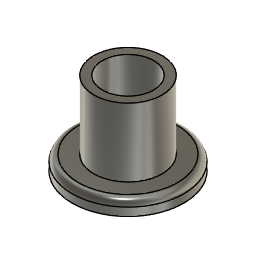
M6x8 socket head sleeve cap v3 (Autodesk Fusion 360 design; units mm, degrees)
Autodesk Fusion 360 part; units mm, degrees
sketch "Sketch1" plane through (0, 0, 0) normal (0, 0, 1) x (1, 0, 0)
  circle A0 centre (0, 0) radius 4
  circle A1 centre (0, 0) radius 3
  circle A2 centre (0, 0) radius 6.55
  dimension "d1" = 8
  dimension "d2" = 6
  dimension "d3" = 13.1
  constraint coincident A0.centre A1.centre
  constraint concentric A0 A2
  measures "d1" diameter of A0
  measures "d2" diameter of A1
  measures "d3" diameter of A2
extrude "Extrude1" add sketch "Sketch1" along normal blind 2.7 makes body 1 at (6.5419, -0.3265, 1.8) makes body 2 at (2.9963, -0.1495, 1.8)
extrude "Extrude2" add 1 faces at (-1.1591, 0.5829, 2.7) along direction (0, 0, 1) blind 1.3 on bodies 2 bodies 2
extrude "Extrude3" add sketch "Sketch1" along normal blind 10.7 contours A0 bodies 1 2
sketch "Sketch2" plane through (0, 0, 0) normal (0, 0, -1) x (1, 0, 0)
  circle A0 centre (0, 0) radius 6.55
  line L0 (-2, 0) -> (2, 0) construction
  line L1 (1, -1.7321) -> (-1, 1.7321) construction
  line L2 (1, 1.7321) -> (-1, -1.7321) construction
  line L3 (-2, -2.5) -> (-2, 2.5) construction
  line L4 (-2, 2.5) -> (2, 2.5) construction
  line L5 (2, 2.5) -> (2, -2.5) construction
  line L6 (2, -2.5) -> (-2, -2.5) construction
  line L7 (-1, -1.7321) -> (-2, -1.1547) construction
  line L8 (-1, 1.7321) -> (-2, 1.1547) construction
  line L9 (-2, -1.1547) -> (-2, 1.1547)
  line L10 (1, -1.7321) -> (2, -1.1547) construction
  line L11 (1, 1.7321) -> (2, 1.1547) construction
  line L12 (-2, -1.1547) -> (0, -2.3094)
  line L13 (0, -2.3094) -> (2, -1.1547)
  line L14 (2, 1.1547) -> (0, 2.3094)
  line L15 (0, 2.3094) -> (-2, 1.1547)
  line L16 (2, -1.1547) -> (2, 1.1547)
  dimension "d10" = 4
  dimension "d12" = 360
  constraint horizontal L0
  constraint midpoint A0.centre L0
  constraint vertical L3
  constraint perpendicular L3 L4
  constraint perpendicular L4 L5
  constraint perpendicular L5 L6
  constraint coincident L3 L7.end
  constraint perpendicular L2 L7
  constraint coincident L3 L8.end
  constraint perpendicular L1 L8
  constraint coincident L5 L10.end
  constraint perpendicular L1 L10
  constraint coincident L5 L11.end
  constraint perpendicular L2 L11
  constraint parallel L7 L12
  constraint perpendicular L1 L13
  constraint perpendicular L2 L14
  constraint parallel L8 L15
  measures "d10" distance of L0.start L0.end
extrude "Extrude4" cut sketch "Sketch2" against normal blind 2 contours L9 L12 L13 L14 L15 L16 bodies 1
chamfer "Chamfer1" distance 0.5 distance2 1.9 6 edges at (-1, 1.7321, 2) (1, 1.7321, 2) (2, 0, 2) (1, -1.7321, 2) (-2, 0, 2) (-1, -1.7321, 2) measured on face at (-1.3333, 1.5396, 0.6667) measured on face at (0.6667, 1.9245, 0.6667) measured on face at (2, 0.3849, 0.6667) measured on face at (1.3333, -1.5396, 0.6667) measured on face at (-2, 0.3849, 0.6667) measured on face at (-0.6667, -1.9245, 0.6667) on bodies 1
chamfer "Chamfer2" distance 0.5 distance2 0.2 6 edges at (2, 0, 0) (1, -1.7321, 0) (-1, -1.7321, 0) (-2, 0, 0) (-1, 1.7321, 0) (1, 1.7321, 0) measured on face at (1.7583, -3.0455, 0) measured on face at (1.7583, -3.0455, 0) measured on face at (1.7583, -3.0455, 0) measured on face at (1.7583, -3.0455, 0) measured on face at (1.7583, -3.0455, 0) measured on face at (1.7583, -3.0455, 0) on bodies 1
chamfer "Chamfer3" distance 1 distance2 2 1 edges at (-6.1067, -2.3686, 0) measured on face at (6.5419, -0.3265, 1.8) on bodies 1
fillet "Fillet1" radius 0.75 1 edges at (-6.1067, -2.3686, 2.7) on bodies 1
